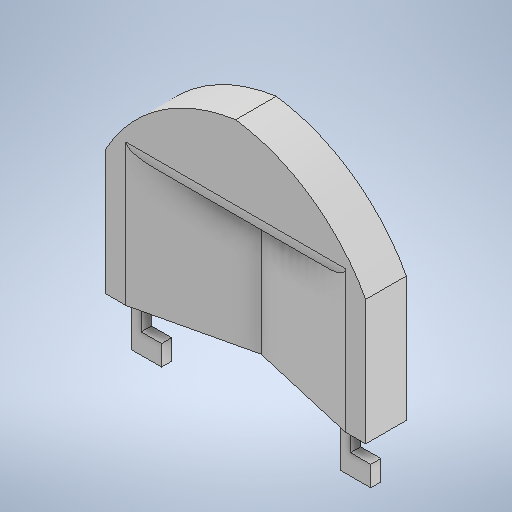
# Autodesk Inventor part: coupole
Saved by Autodesk Inventor 2025.2 (Build 292293000, 293)
## iProperties
Created: 2026-03-12
Part Number: coupole
Material: Générique
Document SubType Name: Modeling
Designer: lcanac
Density: 1 g/cm^3
Appearance: Par défaut
Author: lcanac
Autodesk Inventor part; units mm, degrees
ref_plane "YZ Plane" through (0, 0, 0) normal (1, 0, 0) x (0, 1, 0)
ref_plane "XZ Plane" through (0, 0, 0) normal (0, 1, 0) x (-1, 0, 0)
ref_plane "XY Plane" through (0, 0, 0) normal (0, 0, 1) x (1, 0, 0)
sketch "Esquisse1" plane through (0, 0, 0) normal (0, 0, 1) x (1, 0, 0)
  line L0 (-51.7647, 0) -> (76.2353, 0)
  line L1 (76.2353, 0) -> (76.2353, 106.1647)
  line L2 (76.2353, 106.1647) -> (-51.7647, 106.1647)
  line L3 (-51.7647, 106.1647) -> (-51.7647, 0)
  point P0 (0, 0)
  dimension "d0" = 128
  constraints: 8 end point, 2 parallel, 1 horizontal, 1 perpendicular
  measures "d0" distance between parallel lines of L1 L3
extrude "Extrusion1" add sketch "Esquisse1" along normal blind 20
sketch "Esquisse2" plane through (0, 0, 20) normal (0, 0, 1) x (1, 0, 0)
  line L0 (-51.7647, 106.1647) -> (-51.7647, 0) projected
  line L1 (-51.7647, 61.583) -> (76.7863, 61.583)
  line L2 (76.2353, 106.1647) -> (-51.7647, 106.1647) projected
  arc A0 (76.2353, 61.583) -> (12.2353, 106.1647) centre (0.1874, 20.6401) ccw
  line L3 (-51.7647, 106.1647) -> (-51.7647, 61.583)
  line L4 (-51.7647, 106.1647) -> (76.2353, 106.1647)
  line L5 (76.2353, 0) -> (76.2353, 106.1647) projected
  line L6 (76.2353, 106.1647) -> (76.2353, 61.583)
  arc A1 (12.2353, 106.1647) -> (-51.7647, 61.583) centre (24.2774, 20.6484) ccw
  line L7 (-51.7647, 61.583) -> (-51.7647, 106.1647)
  line L8 (-51.7647, 106.1647) -> (76.2353, 106.1647)
  line L9 (76.2353, 106.1647) -> (76.2353, 61.583)
  point P0 (0, 0)
  dimension "d5" = 86.36
  constraints: 14 end point, 6 collinear, 4 point on circle, 2 centre point, 2 point on line, 1 horizontal, 1 midpoint
  measures "d5" radius of A1
extrude "Extrusion2" cut sketch "Esquisse2" against normal blind 20 contours L2 A1 L0 | L2 L5 A0
sketch "Esquisse3" plane through (-51.7647, 0, 0) normal (0, -1, 0) x (1, 0, 0)
  line L0 (0, 20) -> (128, 20) projected
  line L1 (10, 20) -> (118, 20)
  line L2 (118, 20) -> (118, 7.5)
  line L3 (118, 7.5) -> (10, 7.5)
  line L4 (10, 7.5) -> (10, 20)
  line L5 (0, 0) -> (0, 20) projected
  line L6 (128, 0) -> (128, 20) projected
  line L7 (0, 0) -> (128, 0) projected
  line L8 (10, 20) -> (64, 7.5)
  line L9 (118, 20) -> (64, 7.5)
  line L10 (118, 20) -> (10, 20)
  point P0 (51.7647, 0)
  dimension "d6" = 10
  dimension "d7" = 10
  dimension "d8" = 7.5
  constraints: 14 end point, 2 parallel, 1 collinear, 1 horizontal, 1 midpoint, 1 perpendicular, 1 point on line
  measures "d6" distance between parallel lines of L5 L4
  measures "d7" distance between parallel lines of L6 L2
  measures "d8" distance between parallel lines of L7 L3
extrude "Extrusion3" cut sketch "Esquisse3" against normal blind 60 contours L0 L9 L8
chamfer "Chanfrein1" distance 5.55 angle 45 1 edges at (12.2353, 60, 20)
fillet "Congé1" radius 10 1 edges at (12.2353, 65.55, 20)
sketch "Esquisse4" plane through (-51.7647, 0, 0) normal (0, -1, 0) x (1, 0, 0)
  line L0 (10, 12.5) -> (15, 12.5)
  line L1 (15, 12.5) -> (15, 17.5)
  line L2 (15, 17.5) -> (10, 17.5)
  line L3 (10, 17.5) -> (10, 12.5)
  line L4 (0, 20) -> (10, 20) projected
  line L5 (0, 0) -> (0, 20) projected
  point P0 (51.7647, 0)
  point P1 (5, 20)
  dimension "d15" = 5
  dimension "d16" = 5
  dimension "d17" = 2.5
  dimension "d18" = 10
  constraints: 8 end point, 2 parallel, 1 horizontal, 1 midpoint, 1 perpendicular
  measures "d15" distance of L2.end L1.end
  measures "d16" distance of L0.end L1.end
  measures "d17" distance from line of point (5, 20) L2
  measures "d18" distance between parallel lines of L5 L3
extrude "Extrusion4" add sketch "Esquisse4" along normal blind 20
sketch "Esquisse5" plane through (-36.7647, 0, 17.5) normal (1, 0, 0) x (0, 0, -1)
  point P0 (17.5, 0)
sketch "Esquisse6" plane through (-36.7647, 0, 17.5) normal (1, 0, 0) x (0, 0, -1)
  line L0 (5, 0) -> (5, -20) projected
  line L1 (0, 0) -> (0, -20) projected
  line L2 (5, -20) -> (0, -20)
  line L3 (0, -20) -> (0, -10)
  line L4 (0, -10) -> (5, -10)
  line L5 (5, -10) -> (5, -20)
  point P0 (17.5, 0)
  constraints: 8 end point, 2 parallel, 1 horizontal, 1 midpoint, 1 perpendicular
extrude "Extrusion5" add sketch "Esquisse6" along normal blind 10
sketch "Esquisse7" plane through (-51.7647, 0, 0) normal (0, -1, 0) x (1, 0, 0)
  line L0 (118, 17.5) -> (113, 17.5)
  line L1 (113, 17.5) -> (113, 12.5)
  line L2 (113, 12.5) -> (118, 12.5)
  line L3 (118, 12.5) -> (118, 17.5)
  line L4 (128, 0) -> (128, 20) projected
  line L5 (118, 20) -> (128, 20) projected
  point P0 (51.7647, 0)
  dimension "d23" = 5
  dimension "d24" = 5
  dimension "d25" = 10
  dimension "d26" = 2.5
  constraints: 8 end point, 2 parallel, 1 horizontal, 1 perpendicular
  measures "d23" distance of L2.end L1.end
  measures "d24" distance of L0.end L1.end
  measures "d25" distance between parallel lines of L4 L3
  measures "d26" distance between parallel lines of L5 L0
extrude "Extrusion6" add sketch "Esquisse7" along normal blind 20
sketch "Esquisse8" plane through (66.2353, 0, 17.5) normal (1, 0, 0) x (0, 0, -1)
  line L0 (0, -20) -> (5, -20) projected
  line L1 (5, -10) -> (0, -10) projected
  line L2 (5, -20) -> (0, -20)
  line L3 (0, -20) -> (0, -10)
  line L4 (0, -10) -> (5, -10)
  line L5 (5, -10) -> (5, -20)
  point P0 (17.5, 0)
  constraints: 8 end point, 2 parallel, 1 horizontal, 1 perpendicular
extrude "Extrusion7" add sketch "Esquisse8" along normal blind 10
